Autodesk Fusion 360 part; units mm, degrees
(part 5 of 5)
sketch "Sketch3" plane through (0, 0, 6) normal (0, 0, 1) x (-1, 0, 0)
  arc A0 (-178.1261, -35) -> (-178.4034, -35.084) centre (-178.1261, -35.5) ccw
  line L0 (-178.4034, -35.084) -> (-181.9997, -37.4815)
  arc A1 (-182.277, -37.5655) -> (-181.9997, -37.4815) centre (-182.277, -37.0655) ccw
  line L1 (-182.277, -37.5655) -> (-199.5, -37.5655)
  arc A2 (-200, -37.0655) -> (-199.5, -37.5655) centre (-199.5, -37.0655) ccw
  line L2 (-200, -37.0655) -> (-200, -36.877)
  arc A3 (-199.5, -36.377) -> (-200, -36.877) centre (-199.5, -36.877) ccw
  line L3 (-199.5, -36.377) -> (-182.7168, -36.377)
  arc A4 (-182.7168, -36.377) -> (-182.4395, -36.293) centre (-182.7168, -35.877) ccw
  line L4 (-182.4395, -36.293) -> (-179.126, -34.084)
  arc A5 (-178.8486, -34) -> (-179.126, -34.084) centre (-178.8486, -34.5) ccw
  line L5 (-178.8486, -34) -> (-138.1989, -34)
  line L6 (-138.1989, -34) -> (-135.4453, -29.6006)
  arc A6 (-134.7702, -29.4336) -> (-135.4453, -29.6006) centre (-135.0215, -29.8659) ccw
  line L7 (-134.7702, -29.4336) -> (-134.7335, -29.4549)
  arc A7 (-134.5631, -30.1558) -> (-134.7335, -29.4549) centre (-134.9848, -29.8872) ccw
  line L8 (-134.5631, -30.1558) -> (-137.5017, -34.7686)
  arc A8 (-137.9234, -35) -> (-137.5017, -34.7686) centre (-137.9234, -34.5) ccw
  line L9 (-137.9234, -35) -> (-178.1261, -35)
  line L10 (-187.9341, -32.776) -> (-188.5368, -32.428)
  line L11 (-188.5368, -32.428) -> (-186.3866, -28.7039)
  line L12 (-186.3866, -28.7039) -> (-185.784, -29.0518)
  line L13 (-185.784, -29.0518) -> (-187.9341, -32.776)
  line L14 (-173.3081, -28.7505) -> (-172.7055, -29.0984)
  line L15 (-172.7055, -29.0984) -> (-174.8556, -32.8225)
  line L16 (-174.8556, -32.8225) -> (-175.4582, -32.4746)
  line L17 (-175.4582, -32.4746) -> (-173.3081, -28.7505)
  line L18 (-162.387, -32.5397) -> (-160.2369, -28.8156)
  line L19 (-160.2369, -28.8156) -> (-159.6342, -29.1636)
  line L20 (-159.6342, -29.1636) -> (-161.7843, -32.8877)
  line L21 (-161.7843, -32.8877) -> (-162.387, -32.5397)
  line L22 (-149.3085, -32.5863) -> (-147.1583, -28.8622)
  line L23 (-147.1583, -28.8622) -> (-146.5557, -29.2101)
  line L24 (-146.5557, -29.2101) -> (-148.7058, -32.9343)
  line L25 (-148.7058, -32.9343) -> (-149.3085, -32.5863)
  line L26 (85.3511, -32.7776) -> (79.8251, -35.1458)
  line L27 (79.8251, -35.1458) -> (74.3512, -32.6596)
  line L28 (74.3512, -32.6596) -> (74.3733, -31.6295)
  line L29 (74.3733, -31.6295) -> (79.8362, -34.1107)
  line L30 (79.8362, -34.1107) -> (85.3511, -31.7472)
  line L31 (85.3511, -31.7472) -> (85.3511, -32.7776)
  line L32 (79.9728, -47.0166) -> (74.4988, -44.5304)
  line L33 (74.4988, -44.5304) -> (74.5209, -43.5002)
  line L34 (74.5209, -43.5002) -> (79.9839, -45.9814)
  line L35 (79.9839, -45.9814) -> (85.4987, -43.6179)
  line L36 (85.4987, -43.6179) -> (85.4987, -44.6483)
  line L37 (85.4987, -44.6483) -> (79.9728, -47.0166)
  line L38 (43.8959, -29) -> (65.1857, -29)
  arc A9 (66.0312, -30.534) -> (65.1857, -29) centre (65.1857, -30) ccw
  line L39 (66.0312, -30.534) -> (55.8121, -46.7142)
  arc A10 (54.1413, -46.7449) -> (55.8121, -46.7142) centre (54.9666, -46.1802) ccw
  line L40 (54.1413, -46.7449) -> (43.0706, -30.5647)
  arc A11 (43.8959, -29) -> (43.0706, -30.5647) centre (43.8959, -30) ccw
  line L41 (-147.6405, -32.6135) -> (-145.4904, -28.8894)
  line L42 (-145.4904, -28.8894) -> (-144.8877, -29.2373)
  line L43 (-144.8877, -29.2373) -> (-147.0378, -32.9615)
  line L44 (-147.0378, -32.9615) -> (-147.6405, -32.6135)
  line L45 (-158.5689, -28.8428) -> (-157.9662, -29.1908)
  line L46 (-157.9662, -29.1908) -> (-160.1164, -32.9149)
  line L47 (-160.1164, -32.9149) -> (-160.719, -32.5669)
  line L48 (-160.719, -32.5669) -> (-158.5689, -28.8428)
  line L49 (-171.6401, -28.7777) -> (-171.0375, -29.1256)
  line L50 (-171.0375, -29.1256) -> (-173.1876, -32.8497)
  line L51 (-173.1876, -32.8497) -> (-173.7903, -32.5018)
  line L52 (-173.7903, -32.5018) -> (-171.6401, -28.7777)
  line L53 (-184.116, -29.079) -> (-186.2661, -32.8032)
  line L54 (-186.2661, -32.8032) -> (-186.8688, -32.4552)
  line L55 (-186.8688, -32.4552) -> (-184.7187, -28.7311)
  line L56 (-184.7187, -28.7311) -> (-184.116, -29.079)
  line L57 (-190.302, -32.4589) -> (-188.1519, -28.7348)
  line L58 (-188.1519, -28.7348) -> (-187.5493, -29.0828)
  line L59 (-187.5493, -29.0828) -> (-189.6994, -32.8069)
  line L60 (-189.6994, -32.8069) -> (-190.302, -32.4589)
  line L61 (-176.6209, -32.8535) -> (-177.2235, -32.5055)
  line L62 (-177.2235, -32.5055) -> (-175.0734, -28.7814)
  line L63 (-175.0734, -28.7814) -> (-174.4707, -29.1293)
  line L64 (-174.4707, -29.1293) -> (-176.6209, -32.8535)
  line L65 (-162.0021, -28.8465) -> (-161.3995, -29.1945)
  line L66 (-161.3995, -29.1945) -> (-163.5496, -32.9186)
  line L67 (-163.5496, -32.9186) -> (-164.1523, -32.5707)
  line L68 (-164.1523, -32.5707) -> (-162.0021, -28.8465)
  line L69 (-148.9236, -28.8931) -> (-148.321, -29.2411)
  line L70 (-148.321, -29.2411) -> (-150.4711, -32.9652)
  line L71 (-150.4711, -32.9652) -> (-151.0737, -32.6172)
  line L72 (-151.0737, -32.6172) -> (-148.9236, -28.8931)
  line L73 (79.9842, -42.2409) -> (74.4582, -39.8726)
  line L74 (74.4582, -39.8726) -> (74.4582, -38.8422)
  line L75 (74.4582, -38.8422) -> (79.9731, -41.2057)
  line L76 (79.9731, -41.2057) -> (85.436, -38.7245)
  line L77 (85.436, -38.7245) -> (85.4581, -39.7547)
  line L78 (85.4581, -39.7547) -> (79.9842, -42.2409)
  line L79 (108, 107) -> (105, 107)
  line L80 (105, 107) -> (103, 110)
  line L81 (103, 110) -> (101, 111)
  line L82 (101, 111) -> (98.9961, 113.0039)
  line L83 (98.9961, 113.0039) -> (78.0039, 113.0039)
  line L84 (78.0039, 113.0039) -> (76, 111)
  line L85 (76, 111) -> (58, 111)
  line L86 (58, 111) -> (56, 113)
  line L87 (56, 113) -> (12, 113)
  line L88 (12, 113) -> (10, 111)
  line L89 (10, 111) -> (0, 111)
  line L90 (0, 111) -> (-2, 113)
  line L91 (-2, 113) -> (-195, 113)
  line L92 (-195, 113) -> (-197, 111)
  line L93 (-197, 111) -> (-206, 111)
  line L94 (-206, 111) -> (-208, 113)
  line L95 (-208, 113) -> (-214, 113)
  line L96 (-214, 113) -> (-215, 113)
  line L97 (-215, 113) -> (-221.3805, 106.6195)
  line L98 (-221.3805, 106.6195) -> (-223, 106)
  line L99 (-223, 106) -> (-223, 35)
  line L100 (-223, 35) -> (-222, 34)
  line L101 (-222, 34) -> (-222, 8.6485)
  line L102 (-222, 8.6485) -> (-223, 7)
  line L103 (-223, 7) -> (-223, -36.5124)
  line L104 (-223, -36.5124) -> (-218.7538, -40.3244)
  line L105 (-218.7538, -40.3244) -> (-214.9132, -42.5866)
  line L106 (-214.9132, -42.5866) -> (-209, -42.5866)
  line L107 (-209, -42.5866) -> (-206.5079, -44.8239)
  line L108 (-206.5079, -44.8239) -> (-203, -44.8239)
  line L109 (-203, -44.8239) -> (-198, -49)
  line L110 (-198, -49) -> (-166, -49)
  line L111 (-166, -49) -> (-164.1255, -46.9119)
  line L112 (-164.1255, -46.9119) -> (-144, -46.9119)
  line L113 (-144, -46.9119) -> (-141.6741, -49)
  line L114 (-141.6741, -49) -> (-55, -49)
  line L115 (-55, -49) -> (-53.1255, -46.9119)
  line L116 (-53.1255, -46.9119) -> (-7, -46.9119)
  line L117 (-7, -46.9119) -> (-5, -49)
  line L118 (-5, -49) -> (90.0217, -49)
  line L119 (90.0217, -49) -> (95.0077, -45.5)
  line L120 (95.0077, -45.5) -> (95.0077, -45.4411)
  line L121 (95.0077, -45.4411) -> (94.9816, -37.2145)
  line L122 (94.9816, -37.2145) -> (95, -37.2329)
  line L123 (95, -37.2329) -> (95, -27)
  line L124 (95, -27) -> (97, -25)
  line L125 (97, -25) -> (101, -25)
  line L126 (101, -25) -> (102, -23)
  line L127 (102, -23) -> (104, -23)
  line L128 (104, -23) -> (105, -21)
  line L129 (105, -21) -> (107, -21)
  line L130 (107, -21) -> (108, -19)
  line L131 (108, -19) -> (108, 24)
  line L132 (108, 24) -> (106, 28)
  line L133 (106, 28) -> (106, 58)
  line L134 (106, 58) -> (108, 59)
  line L135 (108, 59) -> (108, 88.6859)
  line L136 (108, 88.6859) -> (106.5, 90)
  line L137 (106.5, 90) -> (106.5, 95)
  line L138 (106.5, 95) -> (108, 96)
  line L139 (108, 96) -> (108, 107)
  line L140 (79.9047, -39.8001) -> (74.4308, -37.3139)
  line L141 (74.4308, -37.3139) -> (74.4529, -36.2838)
  line L142 (74.4529, -36.2838) -> (79.9158, -38.765)
  line L143 (79.9158, -38.765) -> (85.4307, -36.4015)
  line L144 (85.4307, -36.4015) -> (85.4307, -37.4319)
  line L145 (85.4307, -37.4319) -> (79.9047, -39.8001)
  line L146 (-151.3887, -42.0152) -> (-188.2093, -42.0152)
  line L147 (-188.2093, -42.0152) -> (-189.9389, -39.1613)
  line L148 (-189.9389, -39.1613) -> (-153.2344, -39.0462)
  line L149 (-153.2344, -39.0462) -> (-151.3887, -42.0152)
  line L150 (-149.9889, -29.2139) -> (-152.1391, -32.938)
  line L151 (-152.1391, -32.938) -> (-152.7417, -32.59)
  line L152 (-152.7417, -32.59) -> (-150.5916, -28.8659)
  line L153 (-150.5916, -28.8659) -> (-149.9889, -29.2139)
  line L154 (-163.6701, -28.8193) -> (-163.0675, -29.1673)
  line L155 (-163.0675, -29.1673) -> (-165.2176, -32.8914)
  line L156 (-165.2176, -32.8914) -> (-165.8203, -32.5435)
  line L157 (-165.8203, -32.5435) -> (-163.6701, -28.8193)
  line L158 (-178.8915, -32.4783) -> (-176.7414, -28.7542)
  line L159 (-176.7414, -28.7542) -> (-176.1387, -29.1021)
  line L160 (-176.1387, -29.1021) -> (-178.2888, -32.8263)
  line L161 (-178.2888, -32.8263) -> (-178.8915, -32.4783)
  line L162 (-182.5931, -29.0881) -> (-184.7432, -32.8122)
  line L163 (-184.7432, -32.8122) -> (-185.3458, -32.4643)
  line L164 (-185.3458, -32.4643) -> (-183.1957, -28.7401)
  line L165 (-183.1957, -28.7401) -> (-182.5931, -29.0881)
  line L166 (-189.2172, -29.0556) -> (-191.3674, -32.7797)
  line L167 (-191.3674, -32.7797) -> (-191.97, -32.4317)
  line L168 (-191.97, -32.4317) -> (-189.8199, -28.7076)
  line L169 (-189.8199, -28.7076) -> (-189.2172, -29.0556)
  line L170 (-213.9474, 108.8427) -> (98.7226, 108.8427)
  arc A12 (103.7226, 103.8427) -> (98.7226, 108.8427) centre (98.7226, 103.8427) ccw
  line L171 (103.7226, 103.8427) -> (103.7226, -17.4007)
  arc A13 (98.7226, -22.4007) -> (103.7226, -17.4007) centre (98.7226, -17.4007) ccw
  line L172 (98.7226, -22.4007) -> (-213.9474, -22.4007)
  arc A14 (-218.9474, -17.4007) -> (-213.9474, -22.4007) centre (-213.9474, -17.4007) ccw
  line L173 (-218.9474, -17.4007) -> (-218.9474, 103.8427)
  arc A15 (-213.9474, 108.8427) -> (-218.9474, 103.8427) centre (-213.9474, 103.8427) ccw
  line L174 (-171.6647, -32.8588) -> (-172.2673, -32.5108)
  line L175 (-172.2673, -32.5108) -> (-170.1172, -28.7867)
  line L176 (-170.1172, -28.7867) -> (-169.5145, -29.1347)
  line L177 (-169.5145, -29.1347) -> (-171.6647, -32.8588)
  line L178 (-159.1961, -32.576) -> (-157.046, -28.8519)
  line L179 (-157.046, -28.8519) -> (-156.4433, -29.1998)
  line L180 (-156.4433, -29.1998) -> (-158.5934, -32.9239)
  line L181 (-158.5934, -32.9239) -> (-159.1961, -32.576)
  line L182 (-146.1175, -32.6226) -> (-143.9674, -28.8984)
  line L183 (-143.9674, -28.8984) -> (-143.3648, -29.2464)
  line L184 (-143.3648, -29.2464) -> (-145.5149, -32.9705)
  line L185 (-145.5149, -32.9705) -> (-146.1175, -32.6226)
  line L186 (79.9726, -30.3701) -> (74.4467, -28.0018)
  line L187 (74.4467, -28.0018) -> (74.4467, -26.9714)
  line L188 (74.4467, -26.9714) -> (79.9615, -29.335)
  line L189 (79.9615, -29.335) -> (85.4245, -26.8538)
  line L190 (85.4245, -26.8538) -> (85.4466, -27.8839)
  line L191 (85.4466, -27.8839) -> (79.9726, -30.3701)
  line L192 (79.8932, -32.8108) -> (74.4193, -30.3246)
  line L193 (74.4193, -30.3246) -> (74.4414, -29.2945)
  line L194 (74.4414, -29.2945) -> (79.9043, -31.7757)
  line L195 (79.9043, -31.7757) -> (85.4192, -29.4122)
  line L196 (85.4192, -29.4122) -> (85.4192, -30.4426)
  line L197 (85.4192, -30.4426) -> (79.8932, -32.8108)
  line L198 (-143.8469, -32.9977) -> (-144.4496, -32.6498)
  line L199 (-144.4496, -32.6498) -> (-142.2994, -28.9256)
  line L200 (-142.2994, -28.9256) -> (-141.6968, -29.2736)
  line L201 (-141.6968, -29.2736) -> (-143.8469, -32.9977)
  line L202 (-155.378, -28.8791) -> (-154.7753, -29.227)
  line L203 (-154.7753, -29.227) -> (-156.9254, -32.9511)
  line L204 (-156.9254, -32.9511) -> (-157.5281, -32.6032)
  line L205 (-157.5281, -32.6032) -> (-155.378, -28.8791)
  line L206 (-168.4492, -28.8139) -> (-167.8466, -29.1619)
  line L207 (-167.8466, -29.1619) -> (-169.9967, -32.886)
  line L208 (-169.9967, -32.886) -> (-170.5993, -32.538)
  line L209 (-170.5993, -32.538) -> (-168.4492, -28.8139)
  line L210 (-181.5277, -28.7673) -> (-180.9251, -29.1153)
  line L211 (-180.9251, -29.1153) -> (-183.0752, -32.8394)
  line L212 (-183.0752, -32.8394) -> (-183.6779, -32.4915)
  line L213 (-183.6779, -32.4915) -> (-181.5277, -28.7673)
  line L214 (-192.8903, -32.7706) -> (-193.493, -32.4227)
  line L215 (-193.493, -32.4227) -> (-191.3428, -28.6985)
  line L216 (-191.3428, -28.6985) -> (-190.7402, -29.0465)
  line L217 (-190.7402, -29.0465) -> (-192.8903, -32.7706)
  line L218 (-177.6617, -29.0931) -> (-179.8118, -32.8172)
  line L219 (-179.8118, -32.8172) -> (-180.4144, -32.4692)
  line L220 (-180.4144, -32.4692) -> (-178.2643, -28.7451)
  line L221 (-178.2643, -28.7451) -> (-177.6617, -29.0931)
  line L222 (-164.5904, -29.1582) -> (-166.7405, -32.8824)
  line L223 (-166.7405, -32.8824) -> (-167.3432, -32.5344)
  line L224 (-167.3432, -32.5344) -> (-165.1931, -28.8103)
  line L225 (-165.1931, -28.8103) -> (-164.5904, -29.1582)
  line L226 (-151.5119, -29.2048) -> (-153.662, -32.9289)
  line L227 (-153.662, -32.9289) -> (-154.2647, -32.581)
  line L228 (-154.2647, -32.581) -> (-152.1145, -28.8569)
  line L229 (-152.1145, -28.8569) -> (-151.5119, -29.2048)
  line L230 (-151.2264, -40.7236) -> (-152.9, -38.3)
  line L231 (-152.9, -38.3) -> (-180.0146, -38.3)
  line L232 (-180.0146, -38.3) -> (-179.2264, -36.7236)
  line L233 (-179.2264, -36.7236) -> (-140.2264, -36.7236)
  line L234 (-140.2264, -36.7236) -> (-144.2264, -40.7236)
  line L235 (-144.2264, -40.7236) -> (-151.2264, -40.7236)
  line L236 (85.3785, -35.1004) -> (79.9046, -37.5866)
  line L237 (79.9046, -37.5866) -> (74.3786, -35.2183)
  line L238 (74.3786, -35.2183) -> (74.3786, -34.1879)
  line L239 (74.3786, -34.1879) -> (79.8935, -36.5514)
  line L240 (79.8935, -36.5514) -> (85.3564, -34.0702)
  line L241 (85.3564, -34.0702) -> (85.3785, -35.1004)
  line L242 (80.0522, -44.5759) -> (74.5262, -42.2076)
  line L243 (74.5262, -42.2076) -> (74.5262, -41.1772)
  line L244 (74.5262, -41.1772) -> (80.0411, -43.5407)
  line L245 (80.0411, -43.5407) -> (85.504, -41.0595)
  line L246 (85.504, -41.0595) -> (85.5261, -42.0897)
  line L247 (85.5261, -42.0897) -> (80.0522, -44.5759)
  line L248 (-153.1799, -29.1776) -> (-155.33, -32.9017)
  line L249 (-155.33, -32.9017) -> (-155.9326, -32.5538)
  line L250 (-155.9326, -32.5538) -> (-153.7825, -28.8297)
  line L251 (-153.7825, -28.8297) -> (-153.1799, -29.1776)
  line L252 (-168.4085, -32.8552) -> (-169.0112, -32.5072)
  line L253 (-169.0112, -32.5072) -> (-166.8611, -28.7831)
  line L254 (-166.8611, -28.7831) -> (-166.2584, -29.131)
  line L255 (-166.2584, -29.131) -> (-168.4085, -32.8552)
  line L256 (-179.9323, -28.7179) -> (-179.3296, -29.0659)
  line L257 (-179.3296, -29.0659) -> (-181.4798, -32.79)
  line L258 (-181.4798, -32.79) -> (-182.0824, -32.4421)
  line L259 (-182.0824, -32.4421) -> (-179.9323, -28.7179)
  line L260 (-193.0108, -28.6714) -> (-192.4082, -29.0193)
  line L261 (-192.4082, -29.0193) -> (-194.5583, -32.7434)
  line L262 (-194.5583, -32.7434) -> (-195.1609, -32.3955)
  line L263 (-195.1609, -32.3955) -> (-193.0108, -28.6714)
  line L264 (-27.9203, -42.5429) -> (-20.2715, -35.9294)
  line L265 (-20.2715, -35.9294) -> (-20.9736, -35.9199)
  spline S0 degree 2 poles (-20.9736, -35.9199) (-22.267, -35.9022) (-22.2516, -34.7659) knots 0 0 0 1 1 1
  spline S1 degree 2 poles (-22.2516, -34.7659) (-22.2464, -34.3871) (-22.0642, -33.8998) knots 0 0 0 1 1 1
  line L266 (-22.0642, -33.8998) -> (-21.0467, -31.1139)
  line L267 (-21.0467, -31.1139) -> (-24.8808, -31.0616)
  spline S2 degree 2 poles (-24.8808, -31.0616) (-24.4356, -29.5892) (-22.1722, -29.6201) knots 0 0 0 1 1 1
  line L268 (-22.1722, -29.6201) -> (-18.9386, -29.6642)
  spline S3 degree 2 poles (-18.9386, -29.6642) (-17.6083, -29.6823) (-17.6217, -30.6708) knots 0 0 0 1 1 1
  spline S4 degree 2 poles (-17.6217, -30.6708) (-17.6249, -30.9018) (-17.7116, -31.1593) knots 0 0 0 1 1 1
  line L269 (-17.7116, -31.1593) -> (-18.9906, -34.8288)
  line L270 (-18.9906, -34.8288) -> (-14.1094, -30.5986)
  spline S5 degree 2 poles (-14.1094, -30.5986) (-13.1183, -29.7435) (-11.8433, -29.7609) knots 0 0 0 1 1 1
  line L271 (-11.8433, -29.7609) -> (-10.2912, -29.7821)
  line L272 (-10.2912, -29.7821) -> (-14.2061, -40.4013)
  line L273 (-14.2061, -40.4013) -> (-9.0417, -40.4717)
  line L274 (-9.0417, -40.4717) -> (-10.4869, -42.7806)
  line L275 (-10.4869, -42.7806) -> (-16.2426, -42.7021)
  spline S6 degree 2 poles (-16.2426, -42.7021) (-17.8224, -42.6806) (-17.8062, -41.4888) knots 0 0 0 1 1 1
  spline S7 degree 2 poles (-17.8062, -41.4888) (-17.8007, -41.0823) (-17.6086, -40.549) knots 0 0 0 1 1 1
  line L276 (-17.6086, -40.549) -> (-15.2728, -33.9185)
  line L277 (-15.2728, -33.9185) -> (-25.0378, -42.5822)
  line L278 (-25.0378, -42.5822) -> (-27.9203, -42.5429)
  line L279 (-32.371, -34.8589) -> (-31.526, -32.5234)
  line L280 (-31.526, -32.5234) -> (-25.2992, -32.6083)
  line L281 (-25.2992, -32.6083) -> (-26.1442, -34.9438)
  line L282 (-26.1442, -34.9438) -> (-32.371, -34.8589)
  spline S8 degree 2 poles (-51.4669, -39.3111) (-51.4484, -37.9531) (-50.0003, -36.79) knots 0 0 0 1 1 1
  spline S9 degree 2 poles (-50.0003, -36.79) (-49.1314, -36.0904) (-47.3643, -35.2551) knots 0 0 0 1 1 1
  spline S10 degree 2 poles (-47.3643, -35.2551) (-48.0589, -34.0167) (-48.0453, -33.0189) knots 0 0 0 1 1 1
  spline S11 degree 2 poles (-48.0453, -33.0189) (-48.0173, -30.9587) (-45.343, -30.0064) knots 0 0 0 1 1 1
  spline S12 degree 2 poles (-45.343, -30.0064) (-43.4303, -29.3302) (-40.8989, -29.3647) knots 0 0 0 1 1 1
  line L283 (-40.8989, -29.3647) -> (-36.0948, -29.4302)
  line L284 (-36.0948, -29.4302) -> (-39.5592, -38.8636)
  line L285 (-39.5592, -38.8636) -> (-42.8851, -38.8183)
  line L286 (-42.8851, -38.8183) -> (-39.9398, -30.8563)
  line L287 (-39.9398, -30.8563) -> (-40.4109, -30.8499)
  spline S13 degree 2 poles (-40.4109, -30.8499) (-42.0277, -30.8278) (-43.1506, -31.1821) knots 0 0 0 1 1 1
  spline S14 degree 2 poles (-43.1506, -31.1821) (-44.812, -31.7231) (-44.8294, -32.9981) knots 0 0 0 1 1 1
  spline S15 degree 2 poles (-44.8294, -32.9981) (-44.835, -33.4046) (-44.4732, -33.9778) knots 0 0 0 1 1 1
  spline S16 degree 2 poles (-44.4732, -33.9778) (-44.1113, -34.551) (-44.1149, -34.8097) knots 0 0 0 1 1 1
  spline S17 degree 2 poles (-44.1149, -34.8097) (-44.1166, -34.939) (-44.1359, -34.9942) knots 0 0 0 1 1 1
  spline S18 degree 2 poles (-44.1359, -34.9942) (-44.3262, -35.3982) (-45.1537, -35.775) knots 0 0 0 1 1 1
  spline S19 degree 2 poles (-45.1537, -35.775) (-46.2975, -36.3046) (-46.8304, -36.7593) knots 0 0 0 1 1 1
  spline S20 degree 2 poles (-46.8304, -36.7593) (-47.7278, -37.514) (-47.7415, -38.5211) knots 0 0 0 1 1 1
  spline S21 degree 2 poles (-47.7415, -38.5211) (-47.7609, -39.9438) (-45.5898, -39.9734) knots 0 0 0 1 1 1
  line L288 (-45.5898, -39.9734) -> (-34.7806, -40.1208)
  line L289 (-34.7806, -40.1208) -> (-36.2351, -42.4295)
  line L290 (-36.2351, -42.4295) -> (-47.0166, -42.2825)
  spline S22 degree 2 poles (-47.0166, -42.2825) (-49.1415, -42.2536) (-50.1961, -41.6663) knots 0 0 0 1 1 1
  spline S23 degree 2 poles (-50.1961, -41.6663) (-51.4892, -40.9464) (-51.4669, -39.3111) knots 0 0 0 1 1 1
  spline S24 degree 2 poles (-65.8366, -35.3082) (-65.4469, -33.835) (-63.5991, -33.8602) knots 0 0 0 1 1 1
  line L291 (-63.5991, -33.8602) -> (-57.8157, -33.9391)
  spline S25 degree 2 poles (-57.8157, -33.9391) (-58.1178, -33.7317) (-58.3045, -33.1886) knots 0 0 0 1 1 1
  spline S26 degree 2 poles (-58.3045, -33.1886) (-58.4911, -32.6455) (-58.4487, -32.2487) knots 0 0 0 1 1 1
  spline S27 degree 2 poles (-58.4487, -32.2487) (-58.2984, -30.7076) (-57.0577, -29.8467) knots 0 0 0 1 1 1
  spline S28 degree 2 poles (-57.0577, -29.8467) (-55.8729, -29.022) (-53.9973, -29.0383) knots 0 0 0 1 1 1
  spline S29 degree 2 poles (-53.9973, -29.0383) (-51.8167, -29.0495) (-50.6554, -29.9432) knots 0 0 0 1 1 1
  spline S30 degree 2 poles (-50.6554, -29.9432) (-49.622, -30.7335) (-49.6393, -31.9992) knots 0 0 0 1 1 1
  spline S31 degree 2 poles (-49.6393, -31.9992) (-49.6427, -32.2486) (-49.6923, -32.4975) knots 0 0 0 1 1 1
  spline S32 degree 2 poles (-49.6923, -32.4975) (-49.9515, -33.8892) (-51.1079, -34.6681) knots 0 0 0 1 1 1
  spline S33 degree 2 poles (-51.1079, -34.6681) (-52.3389, -35.4922) (-54.3714, -35.4645) knots 0 0 0 1 1 1
  line L292 (-54.3714, -35.4645) -> (-65.8366, -35.3082)
  line L293 (-55.7463, -33.9673) -> (-53.6306, -33.9961)
  line L294 (-53.6306, -33.9961) -> (-52.7669, -31.6424)
  spline S34 degree 2 poles (-52.7669, -31.6424) (-52.6997, -31.4585) (-52.6974, -31.2922) knots 0 0 0 1 1 1
  spline S35 degree 2 poles (-52.6974, -31.2922) (-52.6866, -30.4977) (-54.1648, -30.4775) knots 0 0 0 1 1 1
  spline S36 degree 2 poles (-54.1648, -30.4775) (-54.3403, -30.4751) (-54.4698, -30.4826) knots 0 0 0 1 1 1
  line L295 (-54.4698, -30.4826) -> (-55.7463, -33.9673)
  spline S37 degree 2 poles (-72.9772, -30.4058) (-72.5136, -28.9337) (-70.6936, -28.9585) knots 0 0 0 1 1 1
  line L296 (-70.6936, -28.9585) -> (-67.1921, -29.0062)
  spline S38 degree 2 poles (-67.1921, -29.0062) (-65.6955, -29.0266) (-65.7086, -29.9875) knots 0 0 0 1 1 1
  spline S39 degree 2 poles (-65.7086, -29.9875) (-64.6859, -28.8556) (-63.217, -28.8756) knots 0 0 0 1 1 1
  spline S40 degree 2 poles (-63.217, -28.8756) (-62.1361, -28.8904) (-61.4707, -29.5647) knots 0 0 0 1 1 1
  spline S41 degree 2 poles (-61.4707, -29.5647) (-60.8054, -30.2391) (-60.82, -31.3108) knots 0 0 0 1 1 1
  spline S42 degree 2 poles (-60.82, -31.3108) (-60.8463, -33.2417) (-62.3397, -34.3394) knots 0 0 0 1 1 1
  spline S43 degree 2 poles (-62.3397, -34.3394) (-63.6932, -35.3374) (-65.6703, -35.3104) knots 0 0 0 1 1 1
  line L297 (-65.6703, -35.3104) -> (-70.9455, -35.2385)
  line L298 (-70.9455, -35.2385) -> (-69.1432, -30.4581)
  line L299 (-69.1432, -30.4581) -> (-72.9772, -30.4058)
  line L300 (-67.0636, -33.813) -> (-65.0219, -33.8408)
  line L301 (-65.0219, -33.8408) -> (-64.3458, -31.697)
  spline S44 degree 2 poles (-64.3458, -31.697) (-64.2876, -31.4945) (-64.2854, -31.3282) knots 0 0 0 1 1 1
  spline S45 degree 2 poles (-64.2854, -31.3282) (-64.2744, -30.5245) (-65.845, -30.5031) knots 0 0 0 1 1 1
  line L302 (-65.845, -30.5031) -> (-67.0636, -33.813)
  spline S46 degree 2 poles (-83.7772, -30.2586) (-83.7684, -29.6119) (-83.051, -29.1781) knots 0 0 0 1 1 1
  spline S47 degree 2 poles (-83.051, -29.1781) (-82.4174, -28.7986) (-81.7338, -28.808) knots 0 0 0 1 1 1
  line L303 (-81.7338, -28.808) -> (-78.1954, -28.8562)
  spline S48 degree 2 poles (-78.1954, -28.8562) (-76.7911, -28.8754) (-76.807, -30.0394) knots 0 0 0 1 1 1
  spline S49 degree 2 poles (-76.807, -30.0394) (-76.811, -30.3351) (-76.9358, -30.6753) knots 0 0 0 1 1 1
  line L304 (-76.9358, -30.6753) -> (-78.0207, -33.6636)
  line L305 (-78.0207, -33.6636) -> (-76.0528, -33.6904)
  line L306 (-76.0528, -33.6904) -> (-74.9912, -31.0529)
  spline S50 degree 2 poles (-74.9912, -31.0529) (-74.7233, -30.382) (-73.8641, -30.3937) knots 0 0 0 1 1 1
  line L307 (-73.8641, -30.3937) -> (-72.8848, -30.4071)
  line L308 (-72.8848, -30.4071) -> (-74.1404, -33.7165)
  spline S51 degree 2 poles (-74.1404, -33.7165) (-73.5694, -33.8536) (-73.2198, -34.3066) knots 0 0 0 1 1 1
  spline S52 degree 2 poles (-73.2198, -34.3066) (-72.8702, -34.7595) (-72.8782, -35.3415) knots 0 0 0 1 1 1
  spline S53 degree 2 poles (-72.8782, -35.3415) (-72.8927, -36.404) (-73.8891, -36.9725) knots 0 0 0 1 1 1
  spline S54 degree 2 poles (-73.8891, -36.9725) (-74.7179, -37.4417) (-75.8543, -37.4262) knots 0 0 0 1 1 1
  line L309 (-75.8543, -37.4262) -> (-77.3509, -37.4058)
  line L310 (-77.3509, -37.4058) -> (-76.5442, -35.1622)
  line L311 (-76.5442, -35.1622) -> (-81.6531, -35.0925)
  line L312 (-81.6531, -35.0925) -> (-79.9062, -30.3113)
  line L313 (-79.9062, -30.3113) -> (-83.7772, -30.2586)
  spline S55 degree 2 poles (-96.1293, -30.0902) (-95.6472, -28.6183) (-93.8457, -28.6428) knots 0 0 0 1 1 1
  line L314 (-93.8457, -28.6428) -> (-90.3257, -28.6908)
  spline S56 degree 2 poles (-90.3257, -28.6908) (-88.8014, -28.7116) (-88.8422, -29.672) knots 0 0 0 1 1 1
  spline S57 degree 2 poles (-88.8422, -29.672) (-87.8097, -28.4941) (-86.1005, -28.5174) knots 0 0 0 1 1 1
  spline S58 degree 2 poles (-86.1005, -28.5174) (-84.9826, -28.5327) (-84.2983, -29.1703) knots 0 0 0 1 1 1
  spline S59 degree 2 poles (-84.2983, -29.1703) (-83.5865, -29.8269) (-83.6016, -30.9355) knots 0 0 0 1 1 1
  spline S60 degree 2 poles (-83.6016, -30.9355) (-83.629, -32.9403) (-85.2705, -34.0545) knots 0 0 0 1 1 1
  spline S61 degree 2 poles (-85.2705, -34.0545) (-86.7159, -35.0235) (-88.8039, -34.995) knots 0 0 0 1 1 1
  line L315 (-88.8039, -34.995) -> (-90.7255, -34.9688)
  line L316 (-90.7255, -34.9688) -> (-92.5196, -39.8233)
  line L317 (-92.5196, -39.8233) -> (-95.8825, -39.7774)
  line L318 (-95.8825, -39.7774) -> (-92.3137, -30.1422)
  line L319 (-92.3137, -30.1422) -> (-96.1293, -30.0902)
  line L320 (-90.1972, -33.4976) -> (-87.8506, -33.5296)
  line L321 (-87.8506, -33.5296) -> (-87.1214, -31.5528)
  spline S62 degree 2 poles (-87.1214, -31.5528) (-87.0252, -31.2769) (-87.0222, -31.0552) knots 0 0 0 1 1 1
  spline S63 degree 2 poles (-87.0222, -31.0552) (-87.0138, -30.4362) (-87.7968, -30.2592) knots 0 0 0 1 1 1
  spline S64 degree 2 poles (-87.7968, -30.2592) (-88.0732, -30.2) (-88.9786, -30.1876) knots 0 0 0 1 1 1
  line L322 (-88.9786, -30.1876) -> (-90.1972, -33.4976)
extrude "Extrude3" add sketch "Sketch3" along normal blind 1 separate body contours L264 L265 S0 S1 L266 L267 S2 L268 S3 S4 L269 L270 S5 L271 L272 L273 L274 L275 S6 S7 L276 L277 L278 | L279 L280 L281 L282 | S8 S9 S10 S11 S12 L283 L284 L285 L286 L287 S13 S14 S15 S16 S17 S18 S19 S20 S21 L288 L289 L290 S22 S23 | S24 L291 S37 L296 S38 S39 S40 S41 S42 L297 L298 L299 L307 | L291 S25 S26 S27 S28 S29 S30 S31 S32 S33 L292 S42 S43 | L299 S46 S47 L303 S48 S49 L304 L305 L306 S50 L307 L308 S51 S52 S53 S54 L309 L310 L311 L312 L313 S59 | S46 L313 S55 L314 S56 S57 S58 S59 S60 S61 L315 L316 L317 L318 L319 makes body 5 at (69.0508, 33.1699, 6) makes body 5 at (56.0207, 31.6843, 6) makes body 5 at (92.9739, 34.9628, 6) makes body 4 at (13.2567, 34.7006, 6) makes body 2 at (27.6565, 33.3585, 6) makes body 3 at (38.5313, 33.05, 6)
fillet "Fillet5" radius 1.5 8 edges at (226.3114, -116.2067, 6) (228.9474, -30.7077, 6) (226.3114, 54.7913, 6) (57.6124, 57.4273, 6) (-111.0866, 54.7913, 6) (-113.7226, -30.7077, 6) (-111.0866, -116.2067, 6) (57.6124, -118.8427, 6) on bodies 1
